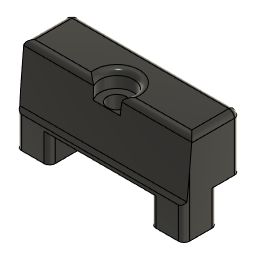
Magnetic Door Clip (Autodesk Fusion 360 design; units mm, degrees)
Autodesk Fusion 360 part; units mm, degrees
note: some values were not read from the file. Chosen so that the rebuilt part matches the saved one: a direction; which face or edge a step refers to; which sketch regions a step uses.
ref_plane "WorkPlane2" through (0, 0, -5.8) normal (0, 0, 1) x (1, 0, 0) in component "Latch"
sketch "facing" plane through (0, 0, -5.8) normal (0, 0, 1) x (1, 0, 0) in component "Latch"
  line L0 (48, 53) -> (78, 53)
  line L1 (72, 47) -> (72, 53)
  line L2 (54, 53) -> (54, 47)
  line L3 (78, 47) -> (48, 47)
  line L4 (48, 47) -> (48, 57)
  line L5 (48, 57) -> (78, 57)
  line L6 (78, 57) -> (78, 47)
  line L7 (108, 50) -> (0, 50) construction
  line L8 (63, 37) -> (63, 67.2217) construction
  circle A0 centre (63, 50) radius 1.7
  circle A1 centre (63, 50) radius 3
  line L9 (64.5, 45.5) -> (61.5, 45.5)
  line L10 (61.5, 45.5) -> (61.5, 48.5)
  line L11 (61.5, 48.5) -> (64.5, 48.5)
  line L12 (64.5, 48.5) -> (64.5, 45.5)
  line L13 (0, 0) -> (0, 105) construction
  dimension "d229" = 10
  dimension "d230" = 3.4
  dimension "d237" = 3
  dimension "d238" = 3
  dimension "d410" = 47
  dimension "d414" = 6
  dimension "d422" = 6
  dimension "d425" = 63
  dimension "d426" = 6
  dimension "latchLength" = 30
  dimension "d431" = 15
  constraint coincident L0 L1.end
  constraint concentric A0 A1
  constraint coincident L13.start origin
  constraint vertical L13
  constraint perpendicular L3 L4
  constraint perpendicular L4 L5
  constraint perpendicular L5 L6
  constraint coincident L0 L2.start
  constraint perpendicular L0 L2
  constraint coincident L0.start L4
  constraint perpendicular L0 L4
  constraint coincident L0.end L6
  constraint perpendicular L1 L3
  constraint coincident L7.end L13
  constraint perpendicular L7 L13
  constraint midpoint L2 L7
  measures "d229" distance of L3.start L5.end
  measures "d230" diameter of A0
  measures "d237" distance of L9.start L9.end
  measures "d238" distance of L9.start L11.end
  measures "d410" distance of L13.start L3
  measures "d414" distance of L3.start L0.end
  measures "d422" distance of L3.start L1.start
  measures "d425" distance of L8 L13
  measures "d426" distance of L2 L4
  measures "latchLength" distance of L4 L6
  measures "d431" distance of L4 L8
extrude "Extrude1" add sketch "facing" against normal blind 6.2 contours L0 L2 L3 L4 | L0 L1 L3 L6 makes body 1 at (72, 49, -7.8667) makes body 2 at (54, 51, -9.9333) in component "Latch"
extrude "Extrude2" add sketch "facing" along normal blind 9.8 contours L0 L4 L5 L6 | L0 L2 L3 L4 | L0 L2 L3 A1 L10 | L0 L1 L3 A1 L12 | A0 A1 L10 L11 L12 | L0 L1 L3 L6 | A0 A1 L10 L11 L12 | L3 A1 L10 | L3 A1 L12 bodies 1 2 in component "Latch"
extrude "Extrude3" add sketch "facing" against normal blind 1.2 contours L0 L2 L3 L4 | L0 L2 L3 A1 L10 | L0 L1 L3 A1 L12 | A0 A1 L10 L11 L12 | L0 L1 L3 L6 | A0 A1 L10 L11 L12 | L3 A1 L10 | L3 A1 L12 bodies 1 in component "Latch"
extrude "Extrude5" cut sketch "facing" against normal blind 3 from surface at 9.8 contours A0 A1 L10 L11 L12 | A0 A1 L10 L11 L12 | L3 A1 L10 | L3 A1 L12 | A0 L11 | A0 L11 bodies 1 in component "Latch"
ref_plane "WorkPlane1" through (0, 47, 0) normal (0, 1, 0) x (0, 0, 1) in component "Latch"
sketch "under" plane through (0, 47, 0) normal (0, 1, 0) x (1, 0, 0) in component "Latch"
  line L0 (48, -4) -> (78, -4)
  line L1 (78, -4) -> (78, 5.8)
  line L2 (78, 5.8) -> (48, 5.8)
  line L3 (48, 5.8) -> (48, -4)
  line L4 (48, 5.8) -> (70, 5.8)
  line L5 (48, -4) -> (48, 12)
  line L6 (78, 5.8) -> (48, 5.8)
  dimension "d266" = 9.8
  dimension "d432" = 30
  constraint horizontal L0
  constraint vertical L1
  constraint horizontal L2
  constraint vertical L3
  constraint horizontal L4
  constraint collinear L4 L6
  constraint collinear L3 L5
  measures "d266" distance of L0 L2
  measures "d432" distance of L1 L3
extrude "Extrude6" cut sketch "under" along normal blind 0.6 bodies 1 in component "Latch"
draft "Draft1" angle 5 neutral plane through (70, 47, -5.8) pull (0, 0, 1) 1 faces at (73.6, 47.6, -0.2667) on bodies 1 in component "Latch"
ref_plane "WorkPlane2" through (0, 0, 4) normal (0, 0, 1) x (1, 0, 0)
sketch "facing (2)" plane through (0, 0, 4) normal (0, 0, 1) x (1, 0, 0) in component "Handle TopBottom"
  line L0 (48, 32) -> (78, 32)
  line L1 (78, 59) -> (48, 59)
  line L2 (48, 59) -> (48, 32)
  line L3 (48, 32) -> (78, 32)
  line L4 (78, 32) -> (78, 46)
  line L5 (78, 46) -> (48, 46)
  line L6 (48, 46) -> (48, 32)
  circle A0 centre (55.5, 35.6) radius 2.35
  circle A1 centre (70.5, 35.6) radius 2.35
  line L7 (48, 35.6) -> (78, 35.6) construction
  circle A2 centre (63, 50) radius 3.05
  line L8 (78, 46) -> (78, 59)
  line L9 (48, 32) -> (78, 59) construction
  line L10 (48, 59) -> (78, 32) construction
  point P0 (63, 45.5)
  dimension "d283" = 27
  dimension "d284" = 30
  dimension "d285" = 14
  dimension "d286" = 4.7
  dimension "d287" = 4.7
  dimension "d288" = 15
  dimension "d289" = 3.6
  dimension "d290" = 7.5
  dimension "d292" = 6.1
  dimension "d293" = 9
  dimension "d294" = 15
  dimension "d305" = 48
  dimension "d306" = 32
  constraint horizontal L0
  constraint horizontal L1
  constraint vertical L2
  constraint horizontal L3
  constraint vertical L4
  constraint horizontal L5
  constraint vertical L6
  constraint coincident L6 L7.start
  constraint coincident L4 L7.end
  constraint perpendicular L4 L7
  constraint coincident A0.centre L7
  constraint coincident A1.centre L7
  constraint perpendicular L1 L8
  constraint midpoint L10 P0
  measures "d283" distance of L0.start L1.end
  measures "d284" distance of L0.start L0.end
  measures "d285" distance of L0.start L5.end
  measures "d286" diameter of A0
  measures "d287" diameter of A1
  measures "d288" horizontal distance of A0.centre A1.centre
  measures "d289" distance of L3 L7
  measures "d290" distance of A0.centre L7.start
  measures "d292" diameter of A2
  measures "d293" distance of L1 A2.centre
  measures "d294" distance of L2 A2.centre
  measures "d305" horizontal distance of origin L0.start
  measures "d306" vertical distance of origin L0.start
extrude "Extrude1'" add sketch "facing (2)" against normal blind 4 separate body contours L0 L2 L3 L4 L5 L6 makes body 3 in component "Handle TopBottom"
extrude "Extrude5'" add sketch "facing (2)" along normal blind 4 contours L0 L2 L3 L4 L5 L6 | L1 L2 L5 L8 | A0 | A1 | A2 bodies 3 in component "Handle TopBottom"
fillet "Fillet3" radius 2 6 edges at (48, 46, 2) (48, 59, 6) (78, 59, 6) (78, 46, 2) (48, 32, 4) (78, 32, 4) on bodies 3 in component "Handle TopBottom"
fillet "Fillet4" radius 2 1 faces at (58.6667, 50, 8) on bodies 3 in component "Handle TopBottom"
extrude "Extrude2'" add sketch "facing (2)" along normal blind 4 contours L0 L2 L3 L4 L5 L6 | A0 | A1 | A2 bodies 3 in component "Handle TopBottom"
extrude "Extrude3'" cut sketch "facing (2)" along normal blind 0.8 contours A0 | A1 bodies 3 in component "Handle TopBottom"
extrude "Extrude4" cut sketch "facing (2)" along normal blind 3 contours A2 bodies 3 in component "Handle TopBottom"
ref_plane "WorkPlane3" through (63, 0, 0) normal (1, 0, 0) x (0, 1, 0)
fillet "Fillet6" radius 2 2 edges at (48, 32, 6) (78, 32, 6) on bodies 3 in component "Handle TopBottom"
fillet "Fillet7" radius 2 5 edges at (48, 40, 8) (48.5858, 32.5858, 8) (63, 32, 8) (77.4142, 32.5858, 8) (78, 40, 8) on bodies 3 in component "Handle TopBottom"
ref_plane "WorkPlane11" through (38, 52, -4) normal (-1, 0, 0) x (0, 1, 0)
mirror "MirrorComponent3" about plane through (0, 0, 0) normal (0, 0, 1) of bodies 3 makes body 4 in component "Handle LeftRight"
sketch "logo topbottom" plane through (0, 0, 8) normal (0, 0, 1) x (1, 0, 0) in component "Handle TopBottom"
  line L0 (57.3646, 38.4891) -> (65.46, 52.5109)
  line L1 (55.0614, 45.5) -> (59.1092, 52.5109)
  line L2 (52, 39.1491) -> (63, 32.7983)
  line L3 (60.54, 38.4891) -> (57.3646, 38.4891)
  line L4 (59.1092, 52.5109) -> (62.2846, 52.5109)
  line L5 (70.9386, 45.5) -> (67.7631, 45.5)
  line L6 (58.2369, 45.5) -> (55.0614, 45.5)
  line L7 (63, 32.7983) -> (74, 39.1491)
  line L8 (74, 39.1491) -> (74, 51.8509)
  line L9 (68.6354, 52.5109) -> (60.54, 38.4891)
  line L10 (52, 51.8509) -> (52, 39.1491)
  line L11 (67.7631, 45.5) -> (63.7154, 38.4891)
  line L12 (63, 45.5) -> (68.5, 55.0263) construction
  line L13 (63.7154, 38.4891) -> (66.8908, 38.4891)
  line L14 (62.2846, 52.5109) -> (58.2369, 45.5)
  line L15 (74, 51.8509) -> (63, 58.2017)
  line L16 (66.8908, 38.4891) -> (70.9386, 45.5)
  line L17 (63, 58.2017) -> (52, 51.8509)
  line L18 (65.46, 52.5109) -> (68.6354, 52.5109)
  line L19 (76, 34) -> (76, 57)
  line L20 (76, 57) -> (50, 57)
  line L21 (50, 57) -> (50, 34)
  line L22 (50, 34) -> (76, 34)
  point P0 (63, 45.5)
  dimension "d462" = 11
  dimension "d463" = 11
  dimension "d464" = 2.75
  dimension "d465" = 0.66
  dimension "d466" = 0.66
  dimension "d467" = 1.375
  dimension "d468" = 2.75
  dimension "d469" = 2.75
  constraint coincident P0 L12.start
  constraint vertical L10
  constraint perpendicular L12 L15
  constraint horizontal L18
  constraint parallel L0 L12
  constraint parallel L0 L9
  constraint parallel L3 L18
  constraint horizontal L4
  constraint parallel L9 L11
  constraint parallel L11 L16
  constraint parallel L0 L14
  constraint parallel L1 L14
  constraint equal L4 L18
  constraint equal L5 L18
  constraint collinear L4 L18
  constraint collinear L3 L13
  constraint parallel L5 L13
  constraint parallel L4 L6
  constraint collinear L5 L6
  constraint equal L11 L14
  measures "d462" distance of P0 L10
  measures "d463" distance of P0 L12.end
  measures "d464" distance of L0 L9
  measures "d465" distance of L8.end L18
  measures "d466" distance of L2.start L3
  measures "d467" distance of L0 L12
  measures "d468" distance of L0 L14
  measures "d469" distance of L9 L11
extrude "Extrude9" cut sketch "logo topbottom" against normal blind 0.8 contours L0 L3 L9 L18 | L1 L4 L6 L14 | L5 L11 L13 L16 bodies 3 in component "Handle TopBottom"
sketch "logo leftright" plane through (0, 0, -8) normal (0, 0, -1) x (1, 0, 0) in component "Handle LeftRight"
  line L0 (76, -57) -> (76, -34)
  line L1 (76, -34) -> (50, -34)
  line L2 (50, -34) -> (50, -57)
  line L3 (50, -57) -> (76, -57)
  line L4 (55.9891, -39.8646) -> (70.0109, -47.96)
  line L5 (55.9891, -49.3908) -> (55.9891, -46.2154)
  line L6 (55.9891, -46.2154) -> (63, -50.2631)
  line L7 (69.3509, -34.5) -> (56.6491, -34.5)
  line L8 (56.6491, -56.5) -> (69.3509, -56.5)
  line L9 (63, -45.5) -> (53.4737, -40) construction
  line L10 (63, -37.5614) -> (63, -40.7369)
  line L11 (70.0109, -41.6092) -> (63, -37.5614)
  line L12 (55.9891, -43.04) -> (55.9891, -39.8646)
  line L13 (69.3509, -56.5) -> (75.7017, -45.5)
  line L14 (63, -40.7369) -> (70.0109, -44.7846)
  line L15 (50.2983, -45.5) -> (56.6491, -56.5)
  line L16 (75.7017, -45.5) -> (69.3509, -34.5)
  line L17 (63, -50.2631) -> (63, -53.4386)
  line L18 (56.6491, -34.5) -> (50.2983, -45.5)
  line L19 (70.0109, -44.7846) -> (70.0109, -41.6092)
  line L20 (63, -53.4386) -> (55.9891, -49.3908)
  line L21 (70.0109, -51.1354) -> (55.9891, -43.04)
  line L22 (70.0109, -47.96) -> (70.0109, -51.1354)
  line L23 (50, -34) -> (76, -57) construction
  line L24 (50, -57) -> (76, -34) construction
  point P0 (63, -45.5)
  point P1 (63, -45.5)
  dimension "d476" = 11
  dimension "d477" = 11
  dimension "d478" = 2.75
  dimension "d479" = 0.66
  dimension "d480" = 0.66
  dimension "d481" = 1.375
  dimension "d482" = 2.75
  dimension "d483" = 2.75
  constraint coincident P1 P0
  constraint perpendicular L9 L18
  constraint parallel L9 L21
  constraint parallel L4 L21
  constraint parallel L12 L22
  constraint parallel L4 L14
  constraint parallel L11 L14
  constraint parallel L6 L21
  constraint parallel L6 L20
  constraint equal L5 L12
  constraint equal L10 L12
  constraint collinear L5 L12
  constraint collinear L19 L22
  constraint parallel L10 L19
  constraint parallel L5 L17
  constraint collinear L10 L17
  constraint equal L6 L14
  constraint coincident L1.end L2.start
  constraint coincident L0.start L3.end
  constraint coincident L2.end L3.start
  constraint coincident L0.end L1.start
  constraint midpoint L23 P1
  measures "d476" distance of P1 L8
  measures "d477" distance of P1 L9.end
  measures "d478" distance of L4 L21
  measures "d479" distance of L7.end L12
  measures "d480" distance of L8.end L22
  measures "d481" distance of L9 L21
  measures "d482" distance of L6 L21
  measures "d483" distance of L4 L14
extrude "Extrude1''" cut sketch "logo leftright" against normal blind 0.8 contours L4 L12 L21 L22 | L5 L6 L17 L20 | L10 L11 L14 L19 bodies 4 in component "Handle LeftRight"
chamfer "Chamfer6" distance 0.6 angle 45 1 edges at (63, 47, -5.8) on bodies 1 in component "Latch"
fillet "Fillet8" radius 1 8 edges at (48, 53, -8.9) (48, 47, -8.9) (54, 47, -9.5) (72, 47, -9.5) (78, 47, -8.9) (78, 53, -8.9) (72, 53, -9.5) (54, 53, -9.5) on bodies 1 in component "Latch"
fillet "Fillet9" radius 1 1 faces at (52.0551, 52.1464, 4) on bodies 1 in component "Latch"
fillet "Fillet10" radius 1 4 edges at (48, 57, -1.4) (48.2929, 56.7071, 3.7071) (78, 57, -1.4) (77.7071, 56.7071, 3.7071) on bodies 1 in component "Latch"
component "Latch" placed x (1, 0, 0) y (0, 1, 0) z (0, 0, 1) at (0, 0, 0)
component "Handle TopBottom" placed x (1, 0, 0) y (0, 1, 0) z (0, 0, 1) at (0, 0, 0)
component "Handle LeftRight" placed x (-1, 0, 0) y (0, 1, 0) z (0, 0, -1) at (76, 0, 0)
equation "FacePlate_height = 40 mm"
equation "thickness = 5.8 mm" comment "Desired thickness usually panel + foam. Consider foam compress to make smaller"
equation "faceThickness = 5 mm" comment "thickness of face, thicker for inserts, thin for tape"
equation "overallThickness = thickness + faceThickness"
equation "screwTrim = max(8 mm - overallThickness; 1 mm)"
equation "d249 = thickness + 4 mm"
equation "d256 = thickness + 4 mm"
equation "capHead = -3 mm"
equation "d266 = thickness + 4 mm"
equation "d281 = -thickness"
equation "d290 = ( d284 - d288 ) / 2"
equation "d328 = 40 mm + 23 mm"
equation "d208 = d140"
equation "d212 = d143 / 2"
equation "d431 = latchLength / 2"
equation "d432 = latchLength"
equation "d209 = d140 * 0.25"
equation "d210 = d140 * 0.06"
equation "d211 = d144"
equation "d213 = d143"
equation "d214 = d143"
equation "d463 = d140"
equation "d464 = d140 * 0.25"
equation "d465 = d140 * 0.06"
equation "d466 = d144"
equation "d467 = d143 / 2"
equation "d468 = d143"
equation "d469 = d143"
equation "d477 = d140"
equation "d478 = d140 * 0.25"
equation "d479 = d140 * 0.06"
equation "d480 = d144"
equation "d481 = d143 / 2"
equation "d482 = d143"
equation "d483 = d143"
